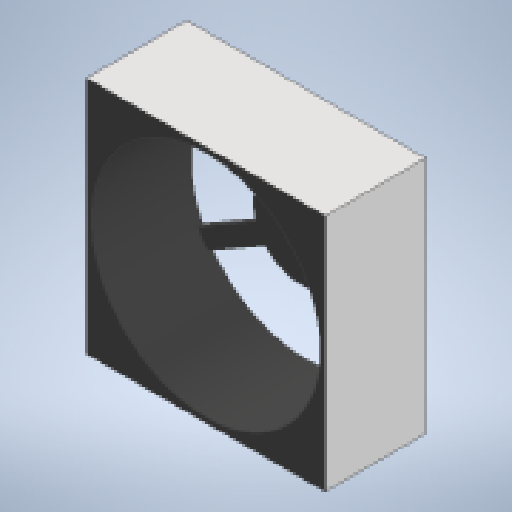
# Autodesk Inventor part: 쿨러
Saved by Autodesk Inventor 2023.1 (Build 271208000, 208)
## iProperties
Created: 2022-08-09
Part Number: 쿨러
Material: 일반
Document SubType Name: Modeling
Designer: fly01
Density: 1 g/cm^3
Appearance: 기본값
Author: fly01
Autodesk Inventor part; units mm, degrees
ref_plane "YZ Plane" through (0, 0, 0) normal (1, 0, 0) x (0, 1, 0)
ref_plane "XZ Plane" through (0, 0, 0) normal (0, 1, 0) x (-1, 0, 0)
ref_plane "XY Plane" through (0, 0, 0) normal (0, 0, 1) x (1, 0, 0)
sketch "스케치1" plane through (0, 0, 0) normal (0, 0, 1) x (1, 0, 0)
  line L0 (-12.5, -12.5) -> (12.5, -12.5)
  line L1 (12.5, -12.5) -> (12.5, 12.5)
  line L2 (12.5, 12.5) -> (-12.5, 12.5)
  line L3 (-12.5, 12.5) -> (-12.5, -12.5)
  line L4 (-12.5, -12.5) -> (12.5, 12.5) construction
  line L5 (12.5, -12.5) -> (-12.5, 12.5) construction
  point P0 (0, 0)
  dimension "d0" = 25
  dimension "d1" = 25
  constraints: 12 end point, 2 midpoint, 2 parallel, 1 horizontal, 1 perpendicular
  measures "d0" distance of L2.end L1.end
  measures "d1" distance of L1.end L0.end
extrude "돌출1" add sketch "스케치1" along normal blind 10.5
sketch "스케치2" plane through (0, 0, 10.5) normal (0, 0, 1) x (1, 0, 0)
  circle A0 centre (0, 0) radius 12
  dimension "d5" = 24
  constraints: 1 centre point, 1 coincident
  measures "d5" diameter of A0
extrude "돌출2" cut sketch "스케치2" against normal blind 10
sketch "스케치3" plane through (0, 0, 0.5) normal (0, 0, 1) x (1, 0, 0)
  circle A0 centre (0, 0) radius 5
  line L0 (-0.9958, 12.5064) -> (1.0042, 12.5064)
  line L1 (1.0042, 12.5064) -> (1.0042, 1.749)
  line L2 (1.0042, 1.749) -> (-0.9958, 1.749)
  line L3 (-0.9958, 1.749) -> (-0.9958, 12.5064)
  line L4 (-0.9958, 12.5064) -> (1.0042, 1.749) construction
  line L5 (1.0042, 12.5064) -> (-0.9958, 1.749) construction
  line L6 (-10.333, -7.1156) -> (-11.333, -5.3835)
  line L7 (-11.333, -5.3835) -> (-2.0168, -0.0048)
  line L8 (-2.0168, -0.0048) -> (-1.0168, -1.7369)
  line L9 (-1.0168, -1.7369) -> (-10.333, -7.1156)
  line L10 (-10.333, -7.1156) -> (-2.0168, -0.0048) construction
  line L11 (-11.333, -5.3835) -> (-1.0168, -1.7369) construction
  line L12 (11.3288, -5.3908) -> (10.3288, -7.1229)
  line L13 (10.3288, -7.1229) -> (1.0126, -1.7442)
  line L14 (1.0126, -1.7442) -> (2.0126, -0.0121)
  line L15 (2.0126, -0.0121) -> (11.3288, -5.3908)
  line L16 (11.3288, -5.3908) -> (1.0126, -1.7442) construction
  line L17 (10.3288, -7.1229) -> (2.0126, -0.0121) construction
  circle A1 centre (0, 0) radius 12 projected
  point P0 (0.0042, 7.1277)
  point P1 (-6.1749, -3.5602)
  point P2 (6.1707, -3.5675)
  point P3 (10.8544, -5.1169)
  point P4 (1.0042, 11.9579)
  point P5 (1.0042, 4.8981)
  point P6 (4.7413, -1.5875)
  point P7 (-9.8586, -6.8417)
  point P8 (9.8537, -6.8486)
  point P9 (3.7398, -3.3187)
  point P10 (-3.7455, -3.3123)
  point P11 (-0.9958, 11.9586)
  point P12 (-10.858, -5.1093)
  point P13 (-4.744, -1.5794)
  point P14 (-0.9958, 4.8998)
  dimension "d8" = 10
  dimension "d11" = 360
  dimension "d13" = 2
  constraints: 36 end point, 2 midpoint, 2 parallel, 1 centre point, 1 coincident, 1 horizontal, 1 perpendicular, 34 other
  measures "d8" diameter of A0
  measures "d13" distance of L1.end L2.end
extrude "돌출3" cut sketch "스케치3" against normal blind 10 contours A0 L1 A1 L15 | A0 L7 A1 L3 | L13 A1 L9 A0
